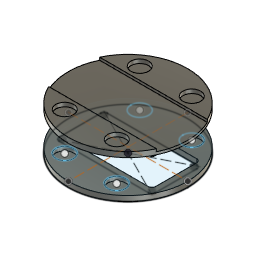
Button holder (Autodesk Fusion 360 design; units mm, degrees)
part number: Wall plate
Autodesk Fusion 360 part; units mm, degrees
sketch "Sketch1" plane through (0, 0, 0) normal (0, 0, 1) x (1, 0, 0) in component "Button"
  circle A0 centre (0, 0) radius 18.15
  line L0 (13.65, 7.35) -> (-13.65, 7.35)
  line L1 (-14.65, 6.35) -> (-14.65, -6.35)
  line L2 (-13.65, -7.35) -> (13.65, -7.35)
  line L3 (14.65, -6.35) -> (14.65, 6.35)
  line L4 (14.65, 7.35) -> (-14.65, -7.35) construction
  line L5 (-14.65, 7.35) -> (14.65, -7.35) construction
  arc A1 (14.65, 6.35) -> (13.65, 7.35) centre (13.65, 6.35) ccw
  arc A2 (13.65, -7.35) -> (14.65, -6.35) centre (13.65, -6.35) ccw
  arc A3 (-14.65, -6.35) -> (-13.65, -7.35) centre (-13.65, -6.35) ccw
  arc A4 (-13.65, 7.35) -> (-14.65, 6.35) centre (-13.65, 6.35) ccw
  dimension "d1" = 36.3
  dimension "d2" = 29.3
  dimension "d3" = 14.7
  dimension "d4" = 1
  dimension "d5" = 1
  dimension "d6" = 1
  dimension "d7" = 1
  constraint coincident A0.centre origin
  constraint horizontal L0
  constraint perpendicular L0 L1
  constraint parallel L0 L2
  constraint parallel L1 L3
  constraint coincident L4 A0.centre
  constraint coincident L5 A0.centre
  constraint coincident L4.start L3
  constraint coincident L4.start L0
  constraint tangent L3 A1
  constraint tangent L0 A1
  constraint coincident L5.end L3
  constraint coincident L5.end L2
  constraint tangent L3 A2
  constraint tangent L2 A2
  constraint coincident L4.end L2
  constraint coincident L4.end L1
  constraint tangent L2 A3
  constraint tangent L1 A3
  constraint coincident L5.start L1
  constraint coincident L5.start L0
  constraint tangent L1 A4
  constraint tangent L0 A4
  measures "d1" diameter of A0
  measures "d2" distance of L4.end L5.end
  measures "d3" distance of L5.start L4.end
  measures "d4" radius of A1
  measures "d5" radius of A2
  measures "d6" radius of A3
  measures "d7" radius of A4
extrude "Extrude1" add sketch "Sketch1" along normal blind 1.6 makes body 1 in component "Button"
sketch "Sketch2" plane through (0, 0, 1.6) normal (0, 0, 1) x (-1, 0, 0) in component "Button"
  arc A0 (13.65, -7.35) -> (14.65, -6.35) centre (13.65, -6.35) ccw
  line L0 (13.65, -7.35) -> (-13.65, -7.35)
  arc A1 (-14.65, -6.35) -> (-13.65, -7.35) centre (-13.65, -6.35) ccw
  line L1 (-14.65, -6.35) -> (-14.65, 6.35)
  arc A2 (-13.65, 7.35) -> (-14.65, 6.35) centre (-13.65, 6.35) ccw
  line L2 (-13.65, 7.35) -> (13.65, 7.35)
  arc A3 (14.65, 6.35) -> (13.65, 7.35) centre (13.65, 6.35) ccw
  line L3 (14.65, 6.35) -> (14.65, -6.35)
  circle A4 centre (0, 0) radius 18.15
  circle A5 centre (7.9215, -11.4948) radius 2.7
  line L4 (0, -18.15) -> (0, 18.15) construction
  line L5 (18.1499, -0.0697) -> (-18.1499, -0.0697) construction
  circle A6 centre (-7.9215, -11.4948) radius 2.7
  circle A7 centre (7.9215, 11.3555) radius 2.7
  circle A8 centre (-7.9215, 11.3555) radius 2.7
  dimension "d10" = 5.4
  constraint coincident A4 L4.start
  constraint coincident A4 L4.end
  constraint perpendicular L2 L4
  constraint coincident A4 L5.start
  constraint coincident A4 L5.end
  constraint perpendicular L1 L5
  constraint symmetric A5 L4 A6
  constraint symmetric A5 L5 A7
  constraint symmetric L5 A6 A8
  measures "d10" diameter of A5
extrude "Extrude2" cut sketch "Sketch2" against normal blind 1.2 contours A5 | A6 | A7 | A8 bodies 1 in component "Button"
copy_body "CutPasteBodies1" bodies 1 removing the originals makes body 2 in component "Button"
ref_plane "WorkPlane1" through (0, 0, 11.6) normal (0, 0, 1) x (-1, 0, 0) in component "Wall plate (1)"
sketch "Sketch3" plane through (0, 0, 11.6) normal (0, 0, 1) x (1, 0, 0) in component "Wall plate (1)"
  circle A0 centre (0, 0) radius 18.15
extrude "Extrude1'" add sketch "Sketch3" along normal blind 1.6 separate body makes body 3 in component "Wall plate (1)"
sketch "Sketch4" plane through (0, 0, 11.6) normal (0, 0, -1) x (1, 0, 0) in component "Wall plate (1)"
  circle A0 centre (0, 0) radius 18.15
  arc A1 (-14.65, -6.35) -> (-13.65, -7.35) centre (-13.65, -6.35) ccw
  line L0 (-14.65, -6.35) -> (-14.65, 6.35)
  arc A2 (-13.65, 7.35) -> (-14.65, 6.35) centre (-13.65, 6.35) ccw
  line L1 (-13.65, 7.35) -> (13.65, 7.35)
  arc A3 (14.65, 6.35) -> (13.65, 7.35) centre (13.65, 6.35) ccw
  line L2 (14.65, 6.35) -> (14.65, -6.35)
  arc A4 (13.65, -7.35) -> (14.65, -6.35) centre (13.65, -6.35) ccw
  line L3 (13.65, -7.35) -> (-13.65, -7.35)
  circle A5 centre (0, 0) radius 18.15
  line L4 (-13.65, 7.15) -> (13.65, 7.15)
  arc A6 (14.45, 6.35) -> (13.65, 7.15) centre (13.65, 6.35) ccw
  line L5 (14.45, 6.35) -> (14.45, -6.35)
  arc A7 (13.65, -7.15) -> (14.45, -6.35) centre (13.65, -6.35) ccw
  line L6 (13.65, -7.15) -> (-13.65, -7.15)
  arc A8 (-14.45, -6.35) -> (-13.65, -7.15) centre (-13.65, -6.35) ccw
  line L7 (-14.45, -6.35) -> (-14.45, 6.35)
  arc A9 (-13.65, 7.15) -> (-14.45, 6.35) centre (-13.65, 6.35) ccw
  dimension "d31" = -0.2
extrude "Extrude2'" add sketch "Sketch4" along normal blind 2 contours L4 A6 L5 A7 L6 A8 L7 A9 bodies 3 in component "Wall plate (1)"
sketch "Sketch5" plane through (0, 0, 13.2) normal (0, 0, 1) x (-1, 0, 0) in component "Wall plate (1)"
  circle A0 centre (0, 0) radius 18.15
  circle A1 centre (-7.9215, 11.3555) radius 2.7
  circle A2 centre (7.9215, 11.3555) radius 2.7
  circle A3 centre (7.9215, -11.4948) radius 2.7
  circle A4 centre (-7.9215, -11.4948) radius 2.7
  line L0 (-23.5, -7.75) -> (23.5, -7.75)
  line L1 (23.5, -7.75) -> (23.5, 7.75)
  line L2 (23.5, 7.75) -> (-23.5, 7.75)
  line L3 (-23.5, 7.75) -> (-23.5, -7.75)
  line L4 (-23.5, -7.75) -> (23.5, 7.75) construction
  line L5 (23.5, -7.75) -> (-23.5, 7.75) construction
  dimension "d36" = 47
  dimension "d37" = 15.5
  constraint horizontal L0
  constraint perpendicular L0 L1
  constraint parallel L0 L2
  constraint parallel L1 L3
  constraint coincident L4 A0.centre
  constraint coincident L5 A0.centre
  constraint coincident A0.centre origin
  measures "d36" distance of L1.end L2.end
  measures "d37" distance of L0.end L1.end
extrude "Extrude3" cut sketch "Sketch5" against normal blind 1.2 contours A1 | A2 | A3 | A4 bodies 3 in component "Wall plate (1)"
extrude "Extrude4" cut sketch "Sketch5" against normal blind 0.8 contours A0 L0 L2 bodies 3 in component "Wall plate (1)"
sketch "Sketch2 (2)" plane through (0, 0, 11.6) normal (0, 0, 1) x (1, 0, 0) in component "Wall plate (1)"
  circle A0 centre (7.9215, 11.4948) radius 2.7
  circle A1 centre (7.9215, -11.3555) radius 2.7
  circle A2 centre (-7.9215, 11.4948) radius 2.7
  circle A3 centre (-7.9215, -11.3555) radius 2.7
  arc A4 (-13.65, 7.35) -> (-14.65, 6.35) centre (-13.65, 6.35) ccw
  line L0 (-13.65, 7.35) -> (13.65, 7.35)
  arc A5 (14.65, 6.35) -> (13.65, 7.35) centre (13.65, 6.35) ccw
  line L1 (14.65, 6.35) -> (14.65, -6.35)
  arc A6 (13.65, -7.35) -> (14.65, -6.35) centre (13.65, -6.35) ccw
  line L2 (13.65, -7.35) -> (-13.65, -7.35)
  arc A7 (-14.65, -6.35) -> (-13.65, -7.35) centre (-13.65, -6.35) ccw
  line L3 (-14.65, -6.35) -> (-14.65, 6.35)
  circle A8 centre (0, 0) radius 18.15
  arc A9 (14.45, 6.35) -> (13.65, 7.15) centre (13.65, 6.35) ccw
  line L4 (-13.65, 7.15) -> (13.65, 7.15)
  arc A10 (-13.65, 7.15) -> (-14.45, 6.35) centre (-13.65, 6.35) ccw
  line L5 (-14.45, -6.35) -> (-14.45, 6.35)
  arc A11 (-14.45, -6.35) -> (-13.65, -7.15) centre (-13.65, -6.35) ccw
  line L6 (13.65, -7.15) -> (-13.65, -7.15)
  arc A12 (13.65, -7.15) -> (14.45, -6.35) centre (13.65, -6.35) ccw
  line L7 (14.45, 6.35) -> (14.45, -6.35)
  dimension "d28" = 0.2
sketch "Sketch1 (2)" plane through (0, 0, 1.6) normal (0, 0, 1) x (-1, 0, 0) in component "Wall plate (1)"
component "Button" placed x (1, 0, 0) y (0, 1, 0) z (0, 0, 1) at (0, 0, 0)
component "Wall plate (1)" placed x (1, 0, 0) y (0, 1, 0) z (0, 0, 1) at (0, 0, 0)
